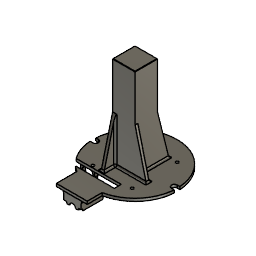
Guide_Stand (Autodesk Fusion 360 design; units mm, degrees)
part number: 2026-04-26-20-37-26-178
Autodesk Fusion 360 part; units mm, degrees
sketch "Sketch1" plane through (0, 0, 0) normal (0, 0, 1) x (1, 0, 0)
  circle A0 centre (0, 0) radius 75
  line L0 (-15, 15) -> (15, 15)
  line L1 (15, 15) -> (15, -15)
  line L2 (15, -15) -> (-15, -15)
  line L3 (-15, -15) -> (-15, 15)
  circle A1 centre (-35, 40) radius 2.5
  circle A2 centre (35, 40) radius 2.5
  circle A3 centre (-35, -40) radius 2.5
  circle A4 centre (35, -40) radius 2.5
  dimension "d1" = 150
  dimension "d2" = 30
  dimension "d3" = 30
  dimension "d4" = 15
  dimension "d5" = 15
  dimension "d6" = 5
  dimension "d7" = 5
  dimension "d8" = 5
  dimension "d9" = 5
  dimension "d10" = 40
  dimension "d11" = 35
  dimension "d12" = 40
  dimension "d13" = 35
  dimension "d14" = 35
  dimension "d15" = 40
  dimension "d16" = 40
  dimension "d17" = 35
  constraint coincident A0.centre origin
  constraint horizontal L0
  constraint vertical L1
  constraint horizontal L2
  constraint vertical L3
  measures "d1" diameter of A0
  measures "d2" distance of L0.start L0.end
  measures "d3" distance of L0.end L1.end
  measures "d4" distance of A0.centre L1
  measures "d5" distance of A0.centre L2
  measures "d6" diameter of A2
  measures "d7" diameter of A1
  measures "d8" diameter of A3
  measures "d9" diameter of A4
  measures "d10" vertical distance of A0.centre A3.centre
  measures "d11" horizontal distance of A0.centre A3.centre
  measures "d12" vertical distance of A0.centre A1.centre
  measures "d13" horizontal distance of A0.centre A1.centre
  measures "d14" horizontal distance of A0.centre A4.centre
  measures "d15" vertical distance of A0.centre A4.centre
  measures "d16" vertical distance of A0.centre A2.centre
  measures "d17" horizontal distance of A0.centre A2.centre
extrude "Extrude17" add sketch "Sketch1" along normal blind 5
sketch "Sketch10" plane through (0, 0, 5) normal (0, 0, 1) x (-1, 0, 0)
  circle A0 centre (-35, 40) radius 2.5
  line L0 (-15, 15) -> (15, 15)
  line L1 (15, 15) -> (15, -15)
  line L2 (15, -15) -> (-15, -15)
  line L3 (-15, -15) -> (-15, 15)
  circle A1 centre (-35, -40) radius 2.5
  circle A2 centre (35, 40) radius 2.5
  circle A3 centre (35, -40) radius 2.5
  circle A4 centre (0, 0) radius 75
  line L4 (15, -15) -> (-15, -15)
  line L5 (-15, -15) -> (-15, 15)
  line L6 (-15, 15) -> (15, 15)
  line L7 (15, 15) -> (15, -15)
  line L8 (20, -20) -> (-20, -20)
  line L9 (-20, -20) -> (-20, 20)
  line L10 (-20, 20) -> (20, 20)
  line L11 (20, 20) -> (20, -20)
  dimension "d81" = 40
  dimension "d82" = 5
  dimension "d83" = 40
  dimension "d84" = 5
  constraint horizontal L4
  constraint vertical L5
  constraint horizontal L6
  constraint vertical L7
  constraint coincident L0.start L3.end
  constraint coincident L1.end L2.start
  constraint horizontal L8
  constraint vertical L9
  constraint horizontal L10
  constraint vertical L11
  measures "d81" distance of L8.start L8.end
  measures "d82" distance of L5 L9
  measures "d83" distance of L8.start L10.end
  measures "d84" distance of L6 L10
extrude "Extrude18" add sketch "Sketch10" along normal blind 157 contours L8 L9 L10 L11
sketch "Sketch11" plane through (0, 0, 162) normal (0, 0, 1) x (-1, 0, 0)
  line L0 (-15, 15) -> (15, 15)
  line L1 (15, 15) -> (15, -15)
  line L2 (15, -15) -> (-15, -15)
  line L3 (-15, -15) -> (-15, 15)
  line L4 (20, 20) -> (-20, 20)
  line L5 (-20, 20) -> (-20, -20)
  line L6 (-20, -20) -> (20, -20)
  line L7 (20, -20) -> (20, 20)
  line L8 (20, -20) -> (-20, -20)
  line L9 (-20, -20) -> (-20, 20)
  line L10 (-20, 20) -> (20, 20)
  line L11 (20, 20) -> (20, -20)
  constraint horizontal L8
  constraint vertical L9
  constraint horizontal L10
  constraint vertical L11
  constraint coincident L4.end L5.start
  constraint coincident L6.end L7.start
extrude "Extrude19" add sketch "Sketch11" along normal blind 5 contours L0 L1 L2 L3 | L4 L5 L6 L7 L8 L9 L10 L11
sketch "Sketch12" plane through (0, 0, 5) normal (0, 0, 1) x (-1, 0, 0)
  line L0 (20, 20) -> (20, -20)
  line L1 (20, -20) -> (-20, -20)
  line L2 (-20, -20) -> (-20, 20)
  line L3 (-20, 20) -> (20, 20)
  circle A0 centre (-35, 40) radius 2.5
  circle A1 centre (-35, -40) radius 2.5
  circle A2 centre (35, 40) radius 2.5
  circle A3 centre (35, -40) radius 2.5
  circle A4 centre (0, 0) radius 75
  line L4 (-20, 20) -> (-40, 20)
  line L5 (-40, 20) -> (-40, 15)
  line L6 (-40, 15) -> (-20, 15)
  line L7 (-20, 15) -> (-20, 20)
  line L8 (20, 20) -> (15, 20)
  line L9 (15, 20) -> (15, 40)
  line L10 (15, 40) -> (20, 40)
  line L11 (20, 40) -> (20, 20)
  line L12 (20, -20) -> (40, -20)
  line L13 (40, -20) -> (40, -15)
  line L14 (40, -15) -> (20, -15)
  line L15 (20, -15) -> (20, -20)
  line L16 (-20, -20) -> (-15, -20)
  line L17 (-15, -20) -> (-15, -40)
  line L18 (-15, -40) -> (-20, -40)
  line L19 (-20, -40) -> (-20, -20)
  dimension "d90" = 20
  dimension "d91" = 5
  dimension "d92" = 5
  dimension "d93" = 20
  dimension "d94" = 5
  dimension "d95" = 20
  dimension "d96" = 20
  dimension "d97" = 5
  constraint horizontal L4
  constraint vertical L5
  constraint horizontal L6
  constraint vertical L7
  constraint coincident L2.end L3.start
  constraint horizontal L8
  constraint vertical L9
  constraint horizontal L10
  constraint vertical L11
  constraint coincident L0.start L3.end
  constraint horizontal L12
  constraint vertical L13
  constraint horizontal L14
  constraint vertical L15
  constraint coincident L0.end L1.start
  constraint horizontal L16
  constraint vertical L17
  constraint horizontal L18
  constraint vertical L19
  constraint coincident L1.end L2.start
  measures "d90" distance of L2.end L4.end
  measures "d91" distance of L4.end L5.end
  measures "d92" distance of L9.end L10.end
  measures "d93" distance of L8.end L9.end
  measures "d94" distance of L0.end L14.end
  measures "d95" distance of L0.end L12.end
  measures "d96" distance of L1.end L18.end
  measures "d97" distance of L1.end L16.end
extrude "Extrude20" add sketch "Sketch12" along normal blind 80 contours L3 L8 L9 L10 L11 | L0 L12 L13 L14 L15 | L2 L4 L5 L6 L7 | L1 L16 L17 L18 L19
sketch "Sketch13" plane through (0, -20, 0) normal (0, -1, 0) x (1, 0, 0)
  line L0 (-20, 85) -> (-15, 85)
  line L1 (-15, 85) -> (-15, 5)
  line L2 (-15, 5) -> (40, 5)
  line L3 (40, 5) -> (40, 85)
  line L4 (40, 85) -> (20, 85)
  line L5 (20, 85) -> (20, 167)
  line L6 (20, 167) -> (-20, 167)
  line L7 (-20, 167) -> (-20, 85)
  line L8 (20, 85) -> (40, 5)
  line L9 (20, 85) -> (40, 85)
  line L10 (40, 5) -> (40, 85)
  constraint coincident L4.end L5.start
  constraint coincident L2.end L3.start
  constraint coincident L3.end L4.start
extrude "Extrude21" cut sketch "Sketch13" against normal blind 5 contours L3 L4 L8 L9 L10
sketch "Sketch14" plane through (-20, 0, 0) normal (-1, 0, 0) x (0, -1, 0)
  line L0 (-20, 85) -> (-15, 85)
  line L1 (-15, 85) -> (-15, 5)
  line L2 (-15, 5) -> (40, 5)
  line L3 (40, 5) -> (40, 85)
  line L4 (40, 85) -> (20, 85)
  line L5 (20, 85) -> (20, 167)
  line L6 (20, 167) -> (-20, 167)
  line L7 (-20, 167) -> (-20, 85)
  line L8 (20, 85) -> (40, 5)
  line L9 (40, 85) -> (20, 85)
  line L10 (40, 85) -> (40, 5)
  constraint coincident L4.end L5.start
  constraint coincident L2.end L3.start
  constraint coincident L3.end L4.start
extrude "Extrude22" cut sketch "Sketch14" against normal blind 5 contours L3 L4 L8 L9 L10
sketch "Sketch15" plane through (0, 20, 0) normal (0, 1, 0) x (-1, 0, 0)
  line L0 (-20, 85) -> (-15, 85)
  line L1 (-15, 85) -> (-15, 5)
  line L2 (-15, 5) -> (40, 5)
  line L3 (40, 5) -> (40, 85)
  line L4 (40, 85) -> (20, 85)
  line L5 (20, 85) -> (20, 167)
  line L6 (20, 167) -> (-20, 167)
  line L7 (-20, 167) -> (-20, 85)
  line L8 (20, 85) -> (40, 5)
  line L9 (40, 85) -> (20, 85)
  line L10 (40, 85) -> (40, 5)
  constraint coincident L4.end L5.start
  constraint coincident L2.end L3.start
  constraint coincident L3.end L4.start
extrude "Extrude23" cut sketch "Sketch15" against normal blind 5 contours L3 L4 L8 L9 L10
sketch "Sketch16" plane through (20, 0, 0) normal (1, 0, 0) x (0, 1, 0)
  line L0 (-15, 85) -> (-15, 5)
  line L1 (-15, 5) -> (40, 5)
  line L2 (40, 5) -> (40, 85)
  line L3 (40, 85) -> (20, 85)
  line L4 (20, 85) -> (20, 167)
  line L5 (20, 167) -> (-20, 167)
  line L6 (-20, 167) -> (-20, 85)
  line L7 (-20, 85) -> (-15, 85)
  line L8 (20, 85) -> (40, 5)
  line L9 (40, 85) -> (40, 5)
  line L10 (20, 85) -> (40, 85)
  constraint coincident L3.end L4.start
  constraint coincident L1.end L2.start
  constraint coincident L2.end L3.start
sketch "Sketch18" plane through (0, 0, 0) normal (0, 0, -1) x (1, 0, 0)
  circle A0 centre (35, 40) radius 2.5
  line L0 (-15, 15) -> (15, 15)
  line L1 (15, 15) -> (15, -15)
  line L2 (15, -15) -> (-15, -15)
  line L3 (-15, -15) -> (-15, 15)
  circle A1 centre (-35, 40) radius 2.5
  circle A2 centre (35, -40) radius 2.5
  circle A3 centre (-35, -40) radius 2.5
  circle A4 centre (0, 0) radius 75
  circle A5 centre (70, 0) radius 5
  circle A6 centre (-70, 0) radius 5
  line L4 (70, -5) -> (74.8331, -5)
  line L5 (70, 5) -> (74.8331, 5)
  line L6 (-70, 5) -> (-74.8331, 5)
  line L7 (-70, -5) -> (-74.8331, -5)
  dimension "d119" = 70
  dimension "d120" = 70
  dimension "d140" = 4.8331
  dimension "d141" = 4.8331
  dimension "d142" = 4.8331
  dimension "d143" = 4.8331
  constraint tangent A4 A5
  constraint tangent A4 A6
  constraint coincident A5 L4.start
  constraint coincident A4 L4.end
  constraint horizontal L4
  constraint coincident A5 L5.start
  constraint coincident A4 L5.end
  constraint parallel L4 L5
  constraint coincident A6 L6.start
  constraint coincident A4 L6.end
  constraint horizontal L6
  constraint coincident A6 L7.start
  constraint coincident A4 L7.end
  constraint parallel L6 L7
  measures "d119" distance of A4.centre A6.centre
  measures "d120" distance of A4.centre A5.centre
  measures "d140" distance of L5.start L5.end
  measures "d141" distance of L4.start L4.end
  measures "d142" distance of L6.start L6.end
  measures "d143" distance of L7.start L7.end
extrude "Extrude31" cut sketch "Sketch16" against normal blind 5 contours L2 L3 L8 L9 L10
extrude "Extrude32" cut sketch "Sketch18" against normal blind 5 contours A4 A5 L5 | A5 | A4 A5 L4 | A4 A6 L6 | A4 A6 L7 | A6
sketch "Sketch21" plane through (0, 0, 0) normal (0, 0, -1) x (1, 0, 0)
  line L0 (74.8331, -5) -> (70, -5)
  arc A0 (70, 5) -> (70, -5) centre (70, 0) ccw
  line L1 (70, 5) -> (74.8331, 5)
  arc A1 (74.8331, 5) -> (-74.8331, 5) centre (0, 0) ccw
  line L2 (-74.8331, 5) -> (-70, 5)
  arc A2 (-70, -5) -> (-70, 5) centre (-70, 0) ccw
  line L3 (-70, -5) -> (-74.8331, -5)
  arc A3 (-74.8331, -5) -> (74.8331, -5) centre (0, 0) ccw
  line L4 (-15, 15) -> (15, 15)
  line L5 (15, 15) -> (15, -15)
  line L6 (15, -15) -> (-15, -15)
  line L7 (-15, -15) -> (-15, 15)
  circle A4 centre (-35, -40) radius 2.5
  circle A5 centre (35, 40) radius 2.5
  circle A6 centre (-35, 40) radius 2.5
  circle A7 centre (35, -40) radius 2.5
  line L8 (0, 75) -> (15, 75)
  line L9 (15, 75) -> (15, 100)
  line L10 (15, 100) -> (0, 100)
  line L11 (0, 100) -> (0, 75)
  line L12 (0, 100) -> (-40, 100)
  line L13 (-40, 100) -> (-40, 75)
  line L14 (-40, 75) -> (0, 75)
  line L15 (0, 75) -> (0, 100)
  line L16 (-40, 75) -> (-40, 63.4429)
  line L17 (15, 75) -> (15, 73.4847)
  dimension "d148" = 25
  dimension "d149" = 15
  dimension "d150" = 40
  constraint horizontal L8
  constraint vertical L9
  constraint horizontal L10
  constraint vertical L11
  constraint midpoint A1 L8.start
  constraint horizontal L12
  constraint vertical L13
  constraint horizontal L14
  constraint vertical L15
  constraint coincident A1 L16.end
  constraint perpendicular L14 L16
  constraint coincident A1 L17.end
  constraint perpendicular L8 L17
  measures "d148" distance of L8.start L10.end
  measures "d149" distance of L9.end L10.end
  measures "d150" distance of L10.end L12.end
extrude "Extrude33" add sketch "Sketch21" against normal blind 5 contours A1 L8 L17 | L8 L9 L10 L11 L15 | L11 L12 L13 L14 L15 | A1 L14 L16
sketch "Sketch23" plane through (0, 0, 5) normal (0, 0, 1) x (-1, 0, 0)
  line L0 (-70, -5) -> (-74.8331, -5)
  arc A0 (-74.8331, -5) -> (74.8331, -5) centre (0, 0) ccw
  line L1 (74.8331, -5) -> (70, -5)
  arc A1 (70, 5) -> (70, -5) centre (70, 0) ccw
  line L2 (70, 5) -> (74.8331, 5)
  arc A2 (74.8331, 5) -> (40, 63.4429) centre (0, 0) ccw
  line L3 (40, 63.4429) -> (40, 100)
  line L4 (40, 100) -> (-15, 100)
  line L5 (-15, 100) -> (-15, 73.4847)
  arc A3 (-15, 73.4847) -> (-74.8331, 5) centre (0, 0) ccw
  line L6 (-74.8331, 5) -> (-70, 5)
  arc A4 (-70, -5) -> (-70, 5) centre (-70, 0) ccw
  line L7 (40, -20) -> (-15, -20)
  line L8 (-15, -20) -> (-15, -40)
  line L9 (-15, -40) -> (-20, -40)
  line L10 (-20, -40) -> (-20, 15)
  line L11 (-20, 15) -> (-40, 15)
  line L12 (-40, 15) -> (-40, 20)
  line L13 (-40, 20) -> (15, 20)
  line L14 (15, 20) -> (15, 40)
  line L15 (15, 40) -> (20, 40)
  line L16 (20, 40) -> (20, -15)
  line L17 (20, -15) -> (40, -15)
  line L18 (40, -15) -> (40, -20)
  circle A5 centre (-35, -40) radius 2.5
  circle A6 centre (35, 40) radius 2.5
  circle A7 centre (-35, 40) radius 2.5
  circle A8 centre (35, -40) radius 2.5
  line L19 (60.7371, 44) -> (-19.2629, 44)
  line L20 (-19.2629, 44) -> (-19.2629, 56)
  line L21 (-19.2629, 56) -> (60.7371, 56)
  line L22 (60.7371, 56) -> (60.7371, 44)
  arc A9 (60.7371, 44) -> (49.8899, 56) centre (0, 0) ccw
  arc A10 (60.7371, 44) -> (49.8899, 56) centre (0, 0) ccw
  point P0 (35, 40)
  dimension "d167" = 12
  dimension "d168" = 4
  dimension "d169" = 80
  constraint horizontal L19
  constraint vertical L20
  constraint horizontal L21
  constraint vertical L22
  constraint coincident A2 L19.start
  constraint coincident A2 A9.end
  constraint coincident L21 A9.end
  measures "d167" distance of L19.start L21.end
  measures "d168" distance of L19 P0
  measures "d169" distance of L20.end L21.end
extrude "Extrude36" cut sketch "Sketch23" against normal blind 5 contours A2 L19 L20 L21 A9 A10
fillet "Fillet1" radius 3 1 edges at (12.5, -20, 5)
fillet "Fillet2" radius 3 11 edges at (-15, -20, 46.5) (-15, -20.8787, 5.8787) (-15, -31.5, 5) (-17.5, -40, 5) (20, 12.5, 5) (30, -15, 5) (40, -19, 5) (17.5, 40, 5) (-40, 17.5, 5) (-12.5, 20, 5) (15, 30, 5)
fillet "Fillet3" radius 3 2 edges at (-31.1712, 15, 5) (-20, -13.6712, 5)
sketch "Sketch24" plane through (0, 0, 5) normal (0, 0, 1) x (-1, 0, 0)
  line L0 (42.3423, -12) -> (42.3423, -23)
  line L1 (42.3423, -23) -> (-12, -23)
  line L2 (-12, -23) -> (-12, -42.3423)
  line L3 (-12, -42.3423) -> (-23, -42.3423)
  line L4 (-23, -42.3423) -> (-23, 12)
  line L5 (-23, 12) -> (-42.3423, 12)
  line L6 (-42.3423, 12) -> (-42.3423, 23)
  line L7 (-42.3423, 23) -> (12, 23)
  line L8 (12, 23) -> (12, 42.3423)
  line L9 (12, 42.3423) -> (23, 42.3423)
  line L10 (23, 42.3423) -> (23, -12)
  line L11 (23, -12) -> (42.3423, -12)
  line L12 (60.7371, 44) -> (-19.2629, 44)
  line L13 (-19.2629, 44) -> (-19.2629, 56)
  line L14 (-19.2629, 56) -> (49.8899, 56)
  arc A0 (49.8899, 56) -> (40, 63.4429) centre (0, 0) ccw
  line L15 (40, 63.4429) -> (40, 100)
  line L16 (40, 100) -> (-15, 100)
  line L17 (-15, 100) -> (-15, 73.4847)
  arc A1 (-15, 73.4847) -> (-74.8331, 5) centre (0, 0) ccw
  line L18 (-74.8331, 5) -> (-70, 5)
  arc A2 (-70, -5) -> (-70, 5) centre (-70, 0) ccw
  line L19 (-70, -5) -> (-74.8331, -5)
  arc A3 (-74.8331, -5) -> (74.8331, -5) centre (0, 0) ccw
  line L20 (74.8331, -5) -> (70, -5)
  arc A4 (70, 5) -> (70, -5) centre (70, 0) ccw
  line L21 (70, 5) -> (74.8331, 5)
  arc A5 (74.8331, 5) -> (60.7371, 44) centre (0, 0) ccw
  circle A6 centre (-35, -40) radius 2.5
  circle A7 centre (35, 40) radius 2.5
  circle A8 centre (-35, 40) radius 2.5
  circle A9 centre (35, -40) radius 2.5
  line L22 (30, 95) -> (0, 95)
  line L23 (0, 95) -> (0, 57)
  line L24 (0, 57) -> (30, 57)
  line L25 (30, 57) -> (30, 95)
  dimension "d178" = 38
  dimension "d179" = 30
  dimension "d180" = 10
  dimension "d181" = 5
  constraint horizontal L22
  constraint vertical L23
  constraint horizontal L24
  constraint vertical L25
  measures "d178" distance of L22.start L24.end
  measures "d179" distance of L22.start L22.end
  measures "d180" distance of L15 L22.start
  measures "d181" distance of L16 L22
sketch "Sketch25" plane through (0, 0, 0) normal (0, 0, -1) x (1, 0, 0)
  line L0 (19.2629, 44) -> (-60.7371, 44)
  arc A0 (-60.7371, 44) -> (-74.8331, 5) centre (0, 0) ccw
  line L1 (-74.8331, 5) -> (-70, 5)
  arc A1 (-70, -5) -> (-70, 5) centre (-70, 0) ccw
  line L2 (-70, -5) -> (-74.8331, -5)
  arc A2 (-74.8331, -5) -> (74.8331, -5) centre (0, 0) ccw
  line L3 (74.8331, -5) -> (70, -5)
  arc A3 (70, 5) -> (70, -5) centre (70, 0) ccw
  line L4 (70, 5) -> (74.8331, 5)
  arc A4 (74.8331, 5) -> (15, 73.4847) centre (0, 0) ccw
  line L5 (15, 73.4847) -> (15, 100)
  line L6 (15, 100) -> (-40, 100)
  line L7 (-40, 100) -> (-40, 63.4429)
  arc A5 (-40, 63.4429) -> (-49.8899, 56) centre (0, 0) ccw
  line L8 (-49.8899, 56) -> (19.2629, 56)
  line L9 (19.2629, 56) -> (19.2629, 44)
  circle A6 centre (35, -40) radius 2.5
  circle A7 centre (-35, 40) radius 2.5
  circle A8 centre (35, 40) radius 2.5
  circle A9 centre (-35, -40) radius 2.5
  line L10 (-15, 15) -> (15, 15)
  line L11 (15, 15) -> (15, -15)
  line L12 (15, -15) -> (-15, -15)
  line L13 (-15, -15) -> (-15, 15)
  line L14 (-33, 95) -> (0, 95)
  line L15 (0, 95) -> (0, 56)
  line L16 (0, 56) -> (-33, 56)
  line L17 (-33, 56) -> (-33, 95)
  dimension "d182" = 39
  dimension "d183" = 5
  dimension "d184" = 33
  dimension "d185" = 7
  constraint horizontal L14
  constraint vertical L15
  constraint horizontal L16
  constraint vertical L17
  measures "d182" distance of L14.start L16.end
  measures "d183" distance of L6 L14
  measures "d184" distance of L14.start L14.end
  measures "d185" distance of L7 L14.start
extrude "Extrude37" add sketch "Sketch25" along normal blind 8.1 contours L8 L14 L15 L16 L17
sketch "Sketch26" plane through (0, 0, -8.1) normal (0, 0, -1) x (1, 0, 0)
  line L0 (-33, 56) -> (0, 56)
  line L1 (0, 56) -> (0, 95)
  line L2 (0, 95) -> (-33, 95)
  line L3 (-33, 95) -> (-33, 56)
  line L4 (-31.7, 93) -> (-30.2, 93)
  line L5 (-30.2, 93) -> (-30.2, 56)
  line L6 (-30.2, 56) -> (-31.7, 56)
  line L7 (-31.7, 56) -> (-31.7, 93)
  line L8 (-2.35, 93) -> (-0.85, 93)
  line L9 (-0.85, 93) -> (-0.85, 56)
  line L10 (-0.85, 56) -> (-2.35, 56)
  line L11 (-2.35, 56) -> (-2.35, 93)
  line L12 (-30, 95) -> (0, 95)
  line L13 (0, 95) -> (0, 57)
  line L14 (-30.2, 57) -> (-2.35, 57)
  line L15 (-2.35, 57) -> (-2.35, 56)
  line L16 (-2.35, 56) -> (-30.2, 56)
  line L17 (-30.2, 56) -> (-30.2, 57)
  dimension "d188" = 37
  dimension "d189" = 2
  dimension "d190" = 1.5
  dimension "d191" = 1.3
  dimension "d192" = 2
  dimension "d194" = 1.5
  dimension "d195" = 37
  dimension "d198" = 27.85
  dimension "d212" = 1
  constraint horizontal L4
  constraint vertical L5
  constraint horizontal L6
  constraint vertical L7
  constraint horizontal L8
  constraint vertical L9
  constraint horizontal L10
  constraint vertical L11
  constraint horizontal L14
  constraint vertical L15
  constraint horizontal L16
  constraint vertical L17
  constraint coincident L5 L14.start
  measures "d188" distance of L4.start L6.end
  measures "d189" distance of L2 L4
  measures "d190" distance of L4.start L4.end
  measures "d191" distance of L3 L7
  measures "d192" distance of L8.start L12
  measures "d194" distance of L8.start L8.end
  measures "d195" distance of L8.end L9.end
  measures "d198" distance of L5.end L10.end
  measures "d212" distance of L14.start L5.end
extrude "Extrude38" add sketch "Sketch26" along normal blind 13.85 contours L0 L4 L5 L6 L7 L17 | L0 L8 L9 L10 L11 L15
sketch "Sketch27" plane through (0, 0, -8.1) normal (0, 0, -1) x (1, 0, 0)
  line L0 (-2.35, 56) -> (-2.35, 93)
  line L1 (-2.35, 93) -> (-0.85, 93)
  line L2 (-0.85, 93) -> (-0.85, 56)
  line L3 (-0.85, 56) -> (0, 56)
  line L4 (-31.7, 56) -> (-31.7, 93)
  line L5 (-31.7, 93) -> (-30.2, 93)
  line L6 (-30.2, 93) -> (-30.2, 56)
  line L7 (0, 56) -> (0, 95)
  line L8 (0, 95) -> (-33, 95)
  line L9 (-33, 95) -> (-33, 56)
  line L10 (-31.7, 95) -> (-0.85, 95)
  line L11 (-0.85, 95) -> (-0.85, 93)
  line L12 (-0.85, 93) -> (-31.7, 93)
  line L13 (-31.7, 93) -> (-31.7, 95)
  line L14 (-33, 56) -> (-31.7, 56)
  line L15 (-30.2, 56) -> (-2.35, 56)
  constraint horizontal L10
  constraint vertical L11
  constraint horizontal L12
  constraint vertical L13
  constraint coincident L1.end L2.start
  constraint coincident L8 L10.start
  constraint coincident L4.end L5.start
extrude "Extrude39" add sketch "Sketch27" along normal blind 13.85 contours L1 L5 L8 L10 L11 L12 L13
sketch "Sketch28" plane through (0, -95, 0) normal (0, -1, 0) x (1, 0, 0)
  line L0 (0, 0) -> (-33, 0)
  line L1 (-33, 0) -> (-33, -8.1)
  line L2 (-33, -8.1) -> (-31.7, -8.1)
  line L3 (-31.7, -8.1) -> (-31.7, -21.95)
  line L4 (-31.7, -21.95) -> (-0.85, -21.95)
  line L5 (-0.85, -21.95) -> (-0.85, -8.1)
  line L6 (-0.85, -8.1) -> (0, -8.1)
  line L7 (0, -8.1) -> (0, 0)
  circle A0 centre (-16.335, -21.95) radius 5
  dimension "d202" = 10
  dimension "d203" = 15.365
  constraint coincident L4 A0.centre
  measures "d202" diameter of A0
  measures "d203" distance of L3.end A0.centre
extrude "Extrude40" cut sketch "Sketch28" against normal blind 2 contours L4 A0 picked at (-14.9579, -20.0286)
sketch "Sketch29" plane through (0, -95, 0) normal (0, -1, 0) x (1, 0, 0)
  arc A0 (-11.335, -21.95) -> (-21.335, -21.95) centre (-16.335, -21.95) ccw
  line L0 (-11.335, -21.95) -> (-0.85, -21.95)
  line L1 (-0.85, -21.95) -> (-0.85, -8.1)
  line L2 (-0.85, -8.1) -> (0, -8.1)
  line L3 (0, -8.1) -> (0, 0)
  line L4 (0, 0) -> (-33, 0)
  line L5 (-33, 0) -> (-33, -8.1)
  line L6 (-31.7, -8.1) -> (-31.7, -21.95)
  line L7 (-31.7, -21.95) -> (-21.335, -21.95)
  line L8 (-0.85, -21.95) -> (-5.85, -21.95)
  line L9 (-5.85, -21.95) -> (-5.85, -18.95)
  line L10 (-5.85, -18.95) -> (-0.85, -18.95)
  line L11 (-0.85, -18.95) -> (-0.85, -21.95)
  line L12 (-31.7, -21.95) -> (-26.7, -21.95)
  line L13 (-26.7, -21.95) -> (-26.7, -18.95)
  line L14 (-26.7, -18.95) -> (-31.7, -18.95)
  line L15 (-31.7, -18.95) -> (-31.7, -21.95)
  line L16 (-33, -8.1) -> (-31.7, -8.1)
  dimension "d206" = 3
  dimension "d207" = 3
  dimension "d208" = 5
  dimension "d209" = 5
  constraint horizontal L8
  constraint vertical L9
  constraint horizontal L10
  constraint vertical L11
  constraint coincident L0.end L1.start
  constraint horizontal L12
  constraint vertical L13
  constraint horizontal L14
  constraint vertical L15
  constraint coincident L6.end L7.start
  measures "d206" distance of L0.end L10.end
  measures "d207" distance of L6.end L14.end
  measures "d208" distance of L0.end L8.end
  measures "d209" distance of L6.end L12.end
extrude "Extrude41" cut sketch "Sketch29" against normal blind 3 contours L0 L1 L8 L9 L10 L11 | L6 L7 L12 L13 L14 L15
sketch "Sketch30" plane through (0, 0, -8.1) normal (0, 0, -1) x (1, 0, 0)
  line L0 (-2.35, 93) -> (-30.2, 93)
  line L1 (-30.2, 93) -> (-30.2, 56)
  line L2 (-30.2, 56) -> (-2.35, 56)
  line L3 (-2.35, 56) -> (-2.35, 93)
extrude "Extrude42" add sketch "Sketch26" along normal blind 5 contours L0 L5 L11 L14 L15 L16 L17
sketch "Sketch32" plane through (0, 0, 0) normal (0, 0, -1) x (1, 0, 0)
  line L0 (0, 95) -> (0, 56)
  line L1 (0, 56) -> (19.2629, 56)
  line L2 (19.2629, 56) -> (19.2629, 44)
  line L3 (19.2629, 44) -> (-60.7371, 44)
  arc A0 (-60.7371, 44) -> (-74.8331, 5) centre (0, 0) ccw
  line L4 (-74.8331, 5) -> (-70, 5)
  arc A1 (-70, -5) -> (-70, 5) centre (-70, 0) ccw
  line L5 (-70, -5) -> (-74.8331, -5)
  arc A2 (-74.8331, -5) -> (74.8331, -5) centre (0, 0) ccw
  line L6 (74.8331, -5) -> (70, -5)
  arc A3 (70, 5) -> (70, -5) centre (70, 0) ccw
  line L7 (70, 5) -> (74.8331, 5)
  arc A4 (74.8331, 5) -> (15, 73.4847) centre (0, 0) ccw
  line L8 (15, 73.4847) -> (15, 100)
  line L9 (15, 100) -> (-40, 100)
  line L10 (-40, 100) -> (-40, 63.4429)
  arc A5 (-40, 63.4429) -> (-49.8899, 56) centre (0, 0) ccw
  line L11 (-49.8899, 56) -> (-33, 56)
  line L12 (-33, 56) -> (-33, 95)
  line L13 (-33, 95) -> (0, 95)
  circle A6 centre (35, -40) radius 2.5
  circle A7 centre (-35, 40) radius 2.5
  circle A8 centre (35, 40) radius 2.5
  circle A9 centre (-35, -40) radius 2.5
  line L14 (-15, 15) -> (15, 15)
  line L15 (15, 15) -> (15, -15)
  line L16 (15, -15) -> (-15, -15)
  line L17 (-15, -15) -> (-15, 15)
  line L18 (-41.835, 24) -> (-66.835, 24)
  line L19 (-66.835, 24) -> (-66.835, 30)
  line L20 (-66.835, 30) -> (-41.835, 30)
  line L21 (-41.835, 30) -> (-41.835, 24)
  line L22 (15, 15) -> (-15, 15)
  dimension "d219" = 26.835
  dimension "d220" = 6
  dimension "d221" = 25
  dimension "d222" = 9
  constraint horizontal L18
  constraint vertical L19
  constraint horizontal L20
  constraint vertical L21
  measures "d219" horizontal distance of L14.start L18.start
  measures "d220" distance of L18.end L19.end
  measures "d221" distance of L18.start L18.end
  measures "d222" distance of L18 L22
extrude "Extrude43" add sketch "Sketch32" along normal blind 21.616 contours L18 L19 L20 L21
sketch "Sketch37" plane through (0, -24, 0) normal (0, 1, 0) x (-1, 0, 0)
  line L0 (66.835, 0) -> (41.835, 0)
  line L1 (41.835, 0) -> (41.835, -21.616)
  line L2 (41.835, -21.616) -> (66.835, -21.616)
  line L3 (66.835, -21.616) -> (66.835, 0)
  circle A0 centre (54.335, -21.616) radius 12.5
  circle A1 centre (54.335, -21.616) radius 9.5
  dimension "d233" = 19
  constraint midpoint L2 A0.centre
  constraint coincident L1.end A0
  constraint concentric A0 A1
  measures "d233" diameter of A1
extrude "Extrude47" add sketch "Sketch37" against normal blind 6 contours L2 A0 A1 picked at (65.7885, -22.237)
extrude "Extrude48" cut sketch "Sketch37" against normal blind 6 contours L2 A1 picked at (54.0984, -18.4582)
fillet "Fillet4" radius 2 4 edges at (-54.335, -24, 0) (-41.835, -27, 0) (-66.835, -27, 0) (-54.335, -30, 0)
fillet "Fillet5" radius 0.5 2 edges at (-45.4779, -24, -18.1807) (-45.4779, -30, -25.0513)
fillet "Fillet6" radius 1 1 edges at (0, -75.5, 0)
fillet "Fillet7" radius 1 4 edges at (-16, -95, 0) (-33, -75.5, 0) (-31.7, -75.5, -8.1) (-0.85, -75.5, -8.1)
chamfer "Chamfer1" distance 0.4 angle 45 2 edges at (-16.335, -95, -16.95) (-16.335, -93, -16.95)
chamfer "Chamfer2" distance 0.5 angle 45 2 edges at (-1.6, -92, -18.95) (-30.95, -92, -18.95)
chamfer "Chamfer3" distance 0.5 angle 45 4 edges at (20, 0, 167) (0, -20, 167) (-20, 0, 167) (0, 20, 167)
chamfer "Chamfer4" distance 1 angle 45 2 edges at (-30.2, -56.5, -13.1) (-2.35, -56.5, -13.1)
chamfer "Chamfer5" distance 0.5 angle 45 2 edges at (-5.85, -94, -18.95) (-26.7, -94, -18.95)
sketch "Sketch38" plane through (0, 0, 0) normal (0, 0, -1) x (1, 0, 0)
  line L0 (-39.835, 32) -> (-39.835, 22)
  line L1 (-39.835, 22) -> (-68.835, 22)
  line L2 (-68.835, 22) -> (-68.835, 29.7782)
  line L3 (-67.8307, 32) -> (-39.835, 32)
  circle A0 centre (35, -40) radius 2.5
  circle A1 centre (-35, 40) radius 2.5
  circle A2 centre (35, 40) radius 2.5
  circle A3 centre (-35, -40) radius 2.5
  line L4 (-15, 15) -> (15, 15)
  line L5 (15, 15) -> (15, -15)
  line L6 (15, -15) -> (-15, -15)
  line L7 (-15, -15) -> (-15, 15)
  line L8 (-34, 56) -> (-34, 96)
  line L9 (-34, 96) -> (1, 96)
  line L10 (1, 96) -> (1, 56)
  line L11 (1, 56) -> (19.2629, 56)
  line L12 (19.2629, 56) -> (19.2629, 44)
  line L13 (19.2629, 44) -> (-60.7371, 44)
  arc A4 (-60.7371, 44) -> (-67.8307, 32) centre (0, 0) ccw
  line L14 (-74.8331, 5) -> (-70, 5)
  arc A5 (-70, -5) -> (-70, 5) centre (-70, 0) ccw
  line L15 (-70, -5) -> (-74.8331, -5)
  arc A6 (-74.8331, -5) -> (74.8331, -5) centre (0, 0) ccw
  line L16 (74.8331, -5) -> (70, -5)
  arc A7 (70, 5) -> (70, -5) centre (70, 0) ccw
  line L17 (70, 5) -> (74.8331, 5)
  arc A8 (74.8331, 5) -> (15, 73.4847) centre (0, 0) ccw
  line L18 (15, 73.4847) -> (15, 100)
  line L19 (15, 100) -> (-40, 100)
  line L20 (-40, 100) -> (-40, 63.4429)
  arc A9 (-40, 63.4429) -> (-49.8899, 56) centre (0, 0) ccw
  line L21 (-49.8899, 56) -> (-34, 56)
  circle A10 centre (0, 0) radius 18
  arc A11 (-68.835, 29.7782) -> (-74.8331, 5) centre (0, 0) ccw
  dimension "d251" = 36
  constraint coincident A4.centre A6.centre
  measures "d251" diameter of A10
extrude "Extrude49" cut sketch "Sketch38" against normal blind 2 contours L4 A10 | L7 A10 | L5 A10 | L6 A10
chamfer "Chamfer6" distance 0.5 angle 45 4 edges at (18, 0, 0) (0, 18, 0) (-18, 0, 0) (0, -18, 0)
equation "d219 = 29.335 mm - 2.5 mm"
